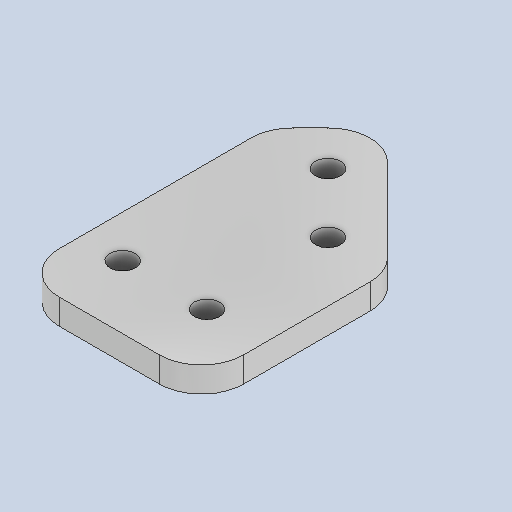
# Autodesk Inventor part: omu_al_jo_5
Saved by Autodesk Inventor 2025.1 (Build 291241000, 241)
## iProperties
Created: 2024-03-23
Part Number: omu_al_jo_5
Material: アルミニウム 6061-AHC
Document SubType Name: Modeling
Designer: fhbdh
Density: 2.7 g/cm^3
Appearance: アルミニウム - ダーク
Author: fhbdh
Autodesk Inventor part; units mm, degrees
ref_plane "YZ Plane" through (0, 0, 0) normal (1, 0, 0) x (0, 1, 0)
ref_plane "XZ Plane" through (0, 0, 0) normal (0, 1, 0) x (-1, 0, 0)
ref_plane "XY Plane" through (0, 0, 0) normal (0, 0, 1) x (1, 0, 0)
derived "omu_sk_jo_1.ipt"
sketch "スケッチ2" plane through (0, 0, 0) normal (0, 1, 0) x (-1, 0, 0)
  line L0 (-340, -340) -> (340, -340) projected
  line L1 (340, -340) -> (340, 340) projected
  line L2 (340, 340) -> (-340, 340) projected
  line L3 (-340, 340) -> (-340, -340) projected
  line L4 (-340, -340) -> (340, 340) construction
  line L5 (340, -340) -> (-340, 340) construction
  line L6 (325, 325) -> (325, -325) projected
  line L7 (325, -325) -> (-325, -325) projected
  line L8 (-325, -325) -> (-325, 325) projected
  line L9 (-325, 325) -> (325, 325) projected
  line L10 (247.2183, 325) -> (325, 247.2183) projected
  line L11 (317.9289, 240.1472) -> (240.1472, 317.9289) projected
  line L12 (240.1472, 317.9289) -> (247.2183, 325) projected
  line L13 (317.9289, 240.1472) -> (325, 247.2183) projected
  line L14 (135.7924, 325) -> (325, 135.7924) projected
  line L15 (325, 135.7924) -> (317.9289, 128.7213) projected
  line L16 (317.9289, 128.7213) -> (128.7213, 317.9289) projected
  line L17 (128.7213, 317.9289) -> (135.7924, 325) projected
  line L18 (243.6827, 321.4645) -> (321.4645, 243.6827) construction
  line L19 (321.4645, 132.2568) -> (132.2568, 321.4645) construction
  line L20 (325, 332.5) -> (-325, 332.5) construction
  line L21 (332.5, 325) -> (332.5, -325) construction
  circle A0 centre (247.2183, 317.9289) radius 1.5 projected
  circle A1 centre (254.2893, 310.8579) radius 1.5 projected
  circle A2 centre (310.8579, 254.2893) radius 1.5 projected
  circle A3 centre (317.9289, 247.2183) radius 1.5 projected
  circle A4 centre (332.5, 257) radius 1.5 projected
  circle A5 centre (332.5, 247) radius 1.5 projected
  circle A6 centre (257, 332.5) radius 1.5 projected
  circle A7 centre (247, 332.5) radius 1.5 projected
  circle A8 centre (135.7924, 317.9289) radius 1.5 projected
  circle A9 centre (142.8634, 310.8579) radius 1.5 projected
  circle A10 centre (145.5741, 332.5) radius 1.5 projected
  circle A11 centre (135.5741, 332.5) radius 1.5 projected
  circle A12 centre (332.5, 145.5741) radius 1.5 projected
  circle A13 centre (332.5, 135.5741) radius 1.5 projected
  circle A14 centre (317.9289, 135.7924) radius 1.5 projected
  circle A15 centre (310.8579, 142.8634) radius 1.5 projected
  line L22 (240.1472, 317.9289) -> (240.1472, 340) projected
  line L23 (262, 340) -> (262, 296.0761) projected
  line L24 (262, 310.2183) -> (254.9289, 303.1472) projected
  circle A16 centre (332.5, 320) radius 1.5 projected
  circle A17 centre (332.5, 310) radius 1.5 projected
  circle A18 centre (320, 332.5) radius 1.5 projected
  circle A19 centre (310, 332.5) radius 1.5 projected
  point P0 (0, 0)
extrude "押し出し1" add sketch "スケッチ2" along normal blind 3 contours L2 L23 L9 L22 | L9 L12 L22 | L23 L10 L9 | L10 L24 L11 L12
fillet "フィレット1" radius 5 5 edges at (-240.1472, 1.5, 340) (-240.1472, 1.5, 317.9289) (-254.9289, 1.5, 303.1472) (-262, 1.5, 310.2183) (-262, 1.5, 340)
